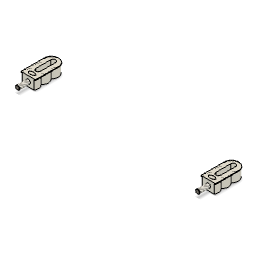
Lamello Cabineo (Autodesk Fusion 360 design; units mm, degrees)
description: Lamello Cabineo
part number: Cabineo
Autodesk Fusion 360 part; units mm, degrees
sketch "Main Sketch" plane through (0, 0, 0) normal (0, 0, 1) x (-1, 0, 0)
  line L0 (160, -9) -> (-160, -9)
  line L1 (-160, -9) -> (-160, 9)
  line L2 (-160, 9) -> (160, 9)
  line L3 (160, 9) -> (160, -9)
  line L4 (160, -9) -> (-160, 9) construction
  line L5 (-160, -9) -> (160, 9) construction
  circle A0 centre (-100, -4) radius 0.5
  circle A1 centre (100, -4) radius 0.5
  dimension "d3" = 320
  dimension "d4" = 18
  dimension "d14" = 1
  dimension "d15" = 1
  dimension "d16" = 60
  dimension "d17" = 60
  dimension "d30" = 13
  dimension "d31" = 13
  constraint horizontal L0
  constraint perpendicular L0 L1
  constraint parallel L0 L2
  constraint parallel L1 L3
  constraint coincident L4 origin
  constraint coincident L5 origin
  measures "d3" distance of L0.start L0.end
  measures "d4" distance of L0 L2
  measures "d14" diameter of A0
  measures "d15" diameter of A1
  measures "d16" distance of L3 A1.centre
  measures "d17" distance of L1 A0.centre
  measures "d30" distance of L2 A1.centre
  measures "d31" distance of L2 A0.centre
extrude "Extrude1" add sketch "Main Sketch" against normal blind 10 contours A0 makes body 1
pattern_linear "R-Pattern1" count 2 spacing 200 along (-1, 0, 0) of bodies 1 makes body 2
sketch "Sketch2" plane through (0, 0, 0) normal (0, 0, 1) x (1, 0, 0)
  circle A0 centre (-100, 4) radius 2.5
  point P0 (-100, 4)
  dimension "d32" = 5
  constraint coincident P0 A0.centre
  measures "d32" diameter of A0
extrude "Extrude2" add sketch "Sketch2" against normal blind 12 separate body makes body 3
ref_plane "WorkPlane1" through (-100, 4, -6) normal (0, 1, 0) x (0, 0, -1)
chamfer "Chamfer1" distance 0.5 angle 45 1 edges at (-102.3308, 4.904, -12) on bodies 3
sketch "Sketch3" plane through (0, 4, 0) normal (0, 1, 0) x (1, 0, 0)
  circle A0 centre (-100, -14.78) radius 7.5
  circle A1 centre (-100, -25.96) radius 7.5
  line L0 (-93.4205, 0) -> (-106.5795, 0)
  line L1 (-160, 0) -> (160, 0)
  arc A2 (-106.5795, 0) -> (-93.4205, 0) centre (-100, -3.6) ccw
  point P0 (-100, 0)
  dimension "d39" = 15
  dimension "d40" = 3.6
  dimension "d41" = 11.18
  dimension "d42" = 11.18
  constraint equal A0 A2
  constraint equal A0 A1
  constraint vertical A2.centre A0.centre
  constraint vertical A2.centre A1.centre
  constraint horizontal L0
  constraint collinear L0 L1
  measures "d39" diameter of A2
  measures "d40" distance of A2.centre P0
  measures "d41" distance of A2.centre A0.centre
  measures "d42" distance of A0.centre A1.centre
extrude "Extrude3" add sketch "Sketch3" along normal mid plane 10 bodies 3
sketch "Sketch4" plane through (0, 9, 0) normal (0, 1, 0) x (-1, 0, 0)
  arc A0 (106.5795, 0) -> (105.0002, 9.19) centre (100, 3.6) ccw
  arc A1 (105.0002, 9.19) -> (105.0002, 20.37) centre (100, 14.78) ccw
  arc A2 (105.0002, 20.37) -> (94.9998, 20.37) centre (100, 25.96) ccw
  arc A3 (94.9998, 20.37) -> (94.9998, 9.19) centre (100, 14.78) ccw
  arc A4 (94.9998, 9.19) -> (93.4205, 0) centre (100, 3.6) ccw
  line L0 (93.4205, 0) -> (106.5795, 0)
  circle A5 centre (100, 25.7) radius 8.1
  line L1 (108.1, 25.7) -> (108.1, 26.442)
  line L2 (108.1, 26.442) -> (108.1, 0)
  line L3 (108.1, 0) -> (91.9, 0)
  line L4 (91.9, 0) -> (91.9, 25.7)
  line L5 (160, 0) -> (-160, 0)
  point P0 (100, 0)
  point P1 (100, 33.8)
  dimension "d47" = 16.2
  dimension "d48" = 33.8
  constraint vertical A5.centre P0
  constraint vertical L1
  constraint horizontal A5.centre L1.start
  constraint horizontal A5.centre L4.end
  constraint tangent A5 L2
  constraint tangent A5 L4
  constraint vertical L4
  constraint collinear L3 L5
  constraint coincident A5 L1.start
  constraint coincident A5 L4.end
  constraint vertical A5.centre P1
  constraint coincident A5 P1
  constraint vertical L2
  measures "d47" diameter of A5
  measures "d48" vertical distance of L3.end P1
extrude "Extrude4" add sketch "Sketch4" 1 faces at (-101.5465, 9, 14.931) along normal blind 0.8 on bodies 3 bodies 3
sketch "Sketch5" plane through (0, 9.8, 0) normal (0, 1, 0) x (-1, 0, 0)
  line L0 (91.9, 0) -> (108.1, 0)
  line L1 (108.1, 0) -> (108.1, 25.7)
  arc A0 (108.1, 25.7) -> (91.9, 25.7) centre (100, 25.7) ccw
  line L2 (91.9, 25.7) -> (91.9, 0)
sketch "Sketch6" plane through (-240, 9.8, 16.9) normal (0, 1, 0) x (-1, 0, 0)
  arc A0 (-144.013, -12.5947) -> (-135.987, -12.5947) centre (-140, -9.6121) ccw
  arc A1 (-135.987, -12.5947) -> (-144.013, -12.5947) centre (-140, -15.5772) ccw
  line L0 (-80, -16.9) -> (-400, -16.9)
  point P0 (-140, -16.9)
  dimension "d77" = 1.3228
  dimension "d78" = 7.2879
  dimension "d79" = 5
  dimension "d80" = 5
  constraint vertical A1.centre P0
  constraint vertical A0.centre P0
  measures "d77" distance of A1.centre L0
  measures "d78" distance of A0.centre L0
  measures "d79" radius of A0
  measures "d80" radius of A1
extrude "Extrude5" add sketch "Sketch6" along normal blind 0.1 bodies 3
sketch "Sketch7" plane through (-240, 9.8, 16.9) normal (0, 1, 0) x (-1, 0, 0)
  line L0 (-137.3, -5.7) -> (-137.3, 10.8)
  arc A0 (-137.3, 10.8) -> (-142.7, 10.8) centre (-140, 10.8) ccw
  line L1 (-142.7, 10.8) -> (-142.7, -5.7)
  arc A1 (-142.7, -5.7) -> (-137.3, -5.7) centre (-140, -5.7) ccw
  line L2 (-140, -5.7) -> (-140, 10.8) construction
  point P0 (-140, -16.9)
  dimension "d53" = 16.5
  dimension "d54" = 2.7
  dimension "d55" = 11.2
  constraint tangent L0 A0
  constraint tangent A0 L1
  constraint parallel L0 L1
  constraint tangent L1 A1
  constraint tangent L0 A1
  constraint vertical L2
  constraint vertical A1.centre P0
  measures "d53" distance of A1.centre A0.centre
  measures "d54" distance of L1 L2
  measures "d55" distance of A1.centre P0
extrude "Extrude6" cut sketch "Sketch7" against normal blind 8 bodies 3
sketch "Sketch8" plane through (0, 4, 0) normal (0, 1, 0) x (1, 0, 0)
  line L0 (-100, -2.6933) -> (-100, -16.5987)
  line L1 (-100, -13) -> (-97, -13)
  line L2 (-97, -13) -> (-97, -8.6)
  line L3 (-97, -8.6) -> (-100, -8.6)
  point P0 (-100, 0)
  dimension "d58" = 6
  dimension "d59" = 4.4
  dimension "d60" = 8.6
  constraint vertical L0
  constraint vertical L0.start P0
  constraint coincident L0 L1.start
  constraint perpendicular L0 L1
  constraint perpendicular L1 L2
  constraint coincident L0 L3.end
  constraint perpendicular L0 L3
  measures "d59" distance of L1 L3
  measures "d60" distance of P0 L3
revolve "Revolve1" add sketch "Sketch8" angle 360 about axis through (-100, 4, 2.6933) along (0, 0, 1) bodies 3
chamfer "Chamfer3" distance 0.2 angle 45 3 edges at (-100, 7, 13) (-97.5886, 2.2154, 13) (-102.4114, 2.2154, 13) on bodies 3
thread "Thread1" "ISO Metric profile 5.0 M5x0.8 6g" major diameter 4.901 minor diameter 3.9895 pitch 0.8 angle 60 resizes the face on face at (-97.5031, 3.8754, -7.6667) on bodies 3
sketch "Sketch9" plane through (-108.1, 0, 0) normal (-1, 0, 0) x (0, 0, 1)
  line L0 (0, 9) -> (25.7, 9)
  line L1 (25.7, 9) -> (25.7, 9.8)
  line L2 (25.7, 9.8) -> (0, 9.8)
  line L3 (0, 9.8) -> (0, 9)
  line L4 (7.94, -2.1651) -> (9.19, 0)
  line L5 (9.19, 0) -> (10.44, -2.1651)
  line L6 (10.44, -2.1651) -> (7.94, -2.1651)
  line L7 (19.12, -2.1651) -> (20.37, 0)
  line L8 (20.37, 0) -> (21.62, -2.1651)
  line L9 (21.62, -2.1651) -> (19.12, -2.1651)
  line L10 (9.19, -1) -> (9.19, 9)
  line L11 (20.37, -1) -> (20.37, 9)
  line L12 (9.19, -1) -> (20.37, -1)
  dimension "d66" = 1
  dimension "d67" = 2.5
  constraint coincident L4.end L10
  constraint coincident L7.end L11
  constraint equal L4 L6
  constraint equal L5 L6
  constraint equal L7 L9
  constraint equal L8 L9
  constraint equal L6 L7
  constraint horizontal L6
  constraint horizontal L9
  constraint horizontal L4.end L7.end
  measures "d66" distance of L4.end L12
  measures "d67" distance of L4.start L5.end
extrude "Extrude7" [suppressed]
copy_body "Body->Comp1" bodies 3 removing the originals makes body 4 in component "Lamello Cabineo"
sketch "Sketch1" plane through (0, 9, 0) normal (0, -1, 0) x (1, 0, 0) in component "Lamello Cabineo"
  arc A0 (-93.4205, 0) -> (-94.9998, 9.19) centre (-100, 3.6) ccw
  line L0 (-93.4205, 0) -> (-91.9, 0)
  line L1 (-91.9, 0) -> (-91.9, 25.7)
  arc A1 (-91.9, 25.7) -> (-108.1, 25.7) centre (-100, 25.7) ccw
  line L2 (-108.1, 25.7) -> (-108.1, 0)
  line L3 (-108.1, 0) -> (-106.5795, 0)
  arc A2 (-105.0002, 9.19) -> (-106.5795, 0) centre (-100, 3.6) ccw
  arc A3 (-105.0002, 20.37) -> (-105.0002, 9.19) centre (-100, 14.78) ccw
  arc A4 (-94.9998, 20.37) -> (-105.0002, 20.37) centre (-100, 25.96) ccw
  arc A5 (-94.9998, 9.19) -> (-94.9998, 20.37) centre (-100, 14.78) ccw
  arc A6 (-94.9998, 20.37) -> (-105.0002, 20.37) centre (-100, 25.96) ccw
  arc A7 (-105.0002, 9.19) -> (-106.5795, 0) centre (-100, 3.6) ccw
  line L4 (-106.5795, 0) -> (-93.4205, 0)
  arc A8 (-93.4205, 0) -> (-94.9998, 9.19) centre (-100, 3.6) ccw
  arc A9 (-94.9998, 9.19) -> (-94.9998, 20.37) centre (-100, 14.78) ccw
  arc A10 (-94.9998, 20.37) -> (-105.0002, 20.37) centre (-100, 25.96) ccw
  arc A11 (-105.0002, 20.37) -> (-105.0002, 9.19) centre (-100, 14.78) ccw
extrude "Extrude1'" add sketch "Sketch1" along normal blind 11 separate body contours A0 A2 A3 A4 A5 A6 A7 L4 A8 A9 A10 A11 makes body 5 in component "Lamello Cabineo"
sketch "Sketch2 (2)" plane through (0, 0, 0) normal (0, 0, -1) x (-1, 0, 0) in component "Lamello Cabineo"
  line L0 (106.5795, -1) -> (106.5795, 9)
  line L1 (106.5795, 9) -> (108.1, 9)
  line L2 (108.1, 9) -> (108.1, 9.8)
  line L3 (108.1, 9.8) -> (91.9, 9.8)
  line L4 (91.9, 9.8) -> (91.9, 9)
  line L5 (91.9, 9) -> (93.4205, 9)
  line L6 (93.4205, 9) -> (93.4205, -1)
  line L7 (93.4205, -1) -> (106.5795, -1)
  circle A0 centre (100, 4) radius 2.4505
  circle A1 centre (100, 4) radius 2.4505
extrude "Extrude2'" add sketch "Sketch2 (2)" along normal blind 12.1 separate body contours A0 A1 makes body 6 in component "Lamello Cabineo"
pattern_linear "00000000-0000-0000-0000-000000000000" [suppressed]
component "Lamello Cabineo" placed x (-1, 0, 0) y (0, 1, 0) z (0, 0, -1) at (0, 0, 0)
component "Lamello Cabineo" placed x (-1, 0, 0) y (0, 1, 0) z (0, 0, -1) at (-200, 0, 0)
hidden bodies 1 2
equation "ContactPatchLength = 320 mm"
equation "ContactPatchWidth = 18.00 mm"
equation "d3 = ContactPatchLength"
equation "d4 = ContactPatchWidth"
equation "MaxDistance = 300 mm"
equation "MinDistance = 20 mm"
equation "UserOffset1 = 60 mm"
equation "UserOffset2 = 60 mm"
equation "PillarBoardT = 18.00 mm"
equation "Coord_Y = ContactPatchWidth - 5 mm"
equation "Offset1 = if(( ContactPatchLength - UserOffset1 - UserOffset2 ) >= MinDistance; UserOffset1; ContactPatchLength / 2)"
equation "Offset2 = if(( ContactPatchLength - UserOffset1 - UserOffset2 ) >= MinDistance; UserOffset2; Offset1)"
equation "d16 = Offset2"
equation "d17 = Offset1"
equation "PlacingLength = ContactPatchLength - Offset1 - Offset2"
equation "NumberOfIntervals = ceil(PlacingLength / MaxDistance)"
equation "NumberOfComponents = if(PlacingLength >= MinDistance; NumberOfIntervals + 1; 1)"
equation "SpaceBetween = if(PlacingLength >= MinDistance; PlacingLength / NumberOfIntervals; 0 mm)"
equation "d26 = NumberOfComponents"
equation "d28 = SpaceBetween"
equation "d30 = Coord_Y"
equation "d31 = Coord_Y"
equation "DrillingDepth = ( if(PillarBoardT <= 16 mm; 8.1; 12.1) ) * 1 mm"
equation "LamelloSize = ( if(PillarBoardT <= 16 mm; 8; 12) ) * 1 mm"
equation "d35 = -LamelloSize"
equation "d42 = d41"
equation "d83 = DrillingDepth"
equation "d89 = NumberOfComponents"
equation "d91 = SpaceBetween"
equation "NestledBoardT = 18 mm"
named bodies: "Lamello Cabineo", "Lamello Cabineo Hole", "Screw Hole"
